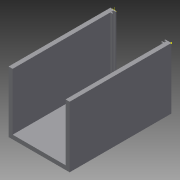
# Autodesk Inventor part: Pièce carré
Saved by Autodesk Inventor 2015 (Build 190159000, 159)
## iProperties
Created: 2015-02-14
Part Number: Pièce carré
Material: Générique
Document SubType Name: Modeling
Designer: informatique
Density: 1 g/cm^3
Appearance: Par défaut
Author: informatique
Autodesk Inventor part; units mm, degrees
ref_plane "YZ Plane" through (0, 0, 0) normal (1, 0, 0) x (0, 1, 0)
sketch "Esquisse1" plane through (0, 0, 0) normal (0, 1, 0) x (-1, 0, 0)
  line L0 (0, 0) -> (30, 0)
  line L1 (30, 0) -> (30, -30)
  line L2 (30, -30) -> (0, -30)
  line L3 (0, -30) -> (0, 0)
  line L4 (28, 0) -> (0, 0)
  line L5 (0, 0) -> (0, -198)
  line L6 (28, 0) -> (2, 0)
  line L7 (2, 0) -> (2, -28)
  line L8 (2, -28) -> (28, -28)
  line L9 (28, -28) -> (28, 0)
  dimension "d0" = 30
  dimension "d1" = 30
  dimension "d4" = 2
  dimension "d5" = 2
  dimension "d6" = 2
  constraints: 20 end point, 4 parallel, 3 horizontal, 3 perpendicular, 2 point on line
  measures "d0" distance of L0.start L0.end
  measures "d1" distance of L2.end L0.start
  measures "d4" distance between parallel lines of L1 L9
  measures "d5" distance between parallel lines of L2 L8
  measures "d6" distance between parallel lines of L3 L7
extrude "Extrusion1" add sketch "Esquisse1" along normal blind 50 contours L0 L7 L8 L9 L1 L2 L3
sketch "Esquisse2" plane through (0, 50, 0) normal (0, 1, 0) x (1, 0, 0)
  point P0 (0, 0)
  point P1 (-28, 0)
  point P2 (-2, 28)
ref_plane "Plan de construction1" through (0, 49.5, 0) normal (0, 1, 0) x (1, 0, 0)
ref_plane "Plan de construction2" through (0, 48, 0) normal (0, 1, 0) x (1, 0, 0)
sketch "Esquisse3" plane through (0, 49.5, 0) normal (0, 1, 0) x (1, 0, 0)
  line L0 (-28, 0) -> (-2, 0)
  line L1 (-2, 0) -> (-2, 28)
  line L2 (-2, 28) -> (-28, 28)
  line L3 (-28, 28) -> (-28, 0)
  line L4 (-27, 0) -> (-3, 0)
  line L5 (-3, 0) -> (-3, 27)
  line L6 (-3, 27) -> (-27, 27)
  line L7 (-27, 27) -> (-27, 0)
  point P0 (0, 0)
  dimension "d14" = 27
  dimension "d15" = 1
  dimension "d16" = 1
  dimension "d17" = 1
  constraints: 16 end point, 4 parallel, 2 horizontal, 2 perpendicular, 1 point on line
  measures "d14" distance of L6.end L4.start
  measures "d15" distance between parallel lines of L3 L7
  measures "d16" distance between parallel lines of L2 L6
  measures "d17" distance between parallel lines of L1 L5
extrude "Extrusion2" add sketch "Esquisse3" along normal blind 0.5 contours L3 L2 L1 L0 L5 L6 L7
sketch "Esquisse4" plane through (0, 48, 0) normal (0, 1, 0) x (1, 0, 0)
  line L0 (-27, 0) -> (-3, 0)
  line L1 (-3, 0) -> (-3, 27)
  line L2 (-3, 27) -> (-27, 27)
  line L3 (-27, 27) -> (-27, 0)
  line L4 (-28, 0) -> (-2, 0)
  line L5 (-2, 0) -> (-2, 28)
  line L6 (-2, 28) -> (-28, 28)
  line L7 (-28, 28) -> (-28, 0)
  point P0 (0, 0)
  constraints: 16 end point, 4 parallel, 2 horizontal, 2 perpendicular
extrude "Extrusion3" add sketch "Esquisse4" along normal blind 0.5 contours L4 L7 L6 L5 L1 L2 L3
